Autodesk Fusion 360 part; units mm, degrees
note: some values were not read from the file. Set by a fixed rule: which sketch regions a step uses.
(part 5 of 8)
sketch "Sketch2" plane through (0, 0, 0) normal (0, 1, 0) x (1, 0, 0)
  spline S0 degree 3 poles (197.1624, -186.7544) (204.143, -186.8486) (204.2626, -186.9263) (213.6388, -187.2436) knots 0 0 0 0 1 1 1 1
  spline S1 degree 3 poles (213.6388, -187.2436) (214.883, -187.1742) (217.6529, -188.4891) (217.5074, -192.0215) knots 0 0 0 0 1 1 1 1
  spline S2 degree 3 poles (217.5074, -192.0215) (217.3575, -195.6649) (214.4757, -196.4537) (213.363, -196.3136) knots 0 0 0 0 1 1 1 1
  spline S3 degree 3 poles (213.363, -196.3136) (204.6057, -196.0144) (204.6194, -195.9201) (197.4444, -195.6721) knots 0 0 0 0 1 1 1 1
  spline S4 degree 3 poles (197.4444, -195.6721) (196.2085, -195.6886) (193.2735, -194.4066) (193.3889, -191.1038) knots 0 0 0 0 1 1 1 1
  spline S5 degree 3 poles (193.3889, -191.1038) (193.5215, -187.3144) (195.7446, -186.8906) (197.1624, -186.7544) knots 0 0 0 0 1 1 1 1
  spline S6 degree 3 poles (197.9086, -187.806) (199.8191, -187.8626) (201.0414, -189.5362) (201.0133, -191.0936) knots 0 0 0 0 1 1 1 1
  spline S7 degree 3 poles (201.0133, -191.0936) (200.9851, -192.7636) (199.4896, -194.3388) (197.734, -194.3215) knots 0 0 0 0 1 1 1 1
  spline S8 degree 3 poles (197.734, -194.3215) (196.0155, -194.305) (194.5332, -192.7609) (194.5124, -190.9876) knots 0 0 0 0 1 1 1 1
  spline S9 degree 3 poles (194.5124, -190.9876) (194.4922, -189.3414) (195.8726, -187.7455) (197.9086, -187.806) knots 0 0 0 0 1 1 1 1
  spline S10 degree 3 poles (197.835, -188.8319) (199.1587, -188.8732) (200.0057, -190.069) (199.9861, -191.1825) knots 0 0 0 0 1 1 1 1
  spline S11 degree 3 poles (199.9861, -191.1825) (199.9618, -192.3766) (198.9303, -193.5028) (197.7139, -193.4905) knots 0 0 0 0 1 1 1 1
  spline S12 degree 3 poles (197.7139, -193.4905) (196.5233, -193.4781) (195.4961, -192.3747) (195.4817, -191.1067) knots 0 0 0 0 1 1 1 1
  spline S13 degree 3 poles (195.4817, -191.1067) (195.4655, -189.9298) (196.4241, -188.7887) (197.835, -188.8319) knots 0 0 0 0 1 1 1 1
  spline S14 degree 3 poles (212.9182, -188.6603) (214.8287, -188.7169) (216.051, -190.3905) (216.0229, -191.9479) knots 0 0 0 0 1 1 1 1
  spline S15 degree 3 poles (216.0229, -191.9479) (215.9947, -193.6179) (214.4992, -195.1931) (212.7436, -195.1758) knots 0 0 0 0 1 1 1 1
  spline S16 degree 3 poles (212.7436, -195.1758) (211.0251, -195.1593) (209.5428, -193.6152) (209.522, -191.8419) knots 0 0 0 0 1 1 1 1
  spline S17 degree 3 poles (209.522, -191.8419) (209.5017, -190.1957) (210.8822, -188.5998) (212.9182, -188.6603) knots 0 0 0 0 1 1 1 1
  spline S18 degree 3 poles (212.8446, -189.6862) (214.1683, -189.7275) (215.0153, -190.9233) (214.9957, -192.0368) knots 0 0 0 0 1 1 1 1
  spline S19 degree 3 poles (214.9957, -192.0368) (214.9714, -193.2309) (213.9399, -194.3572) (212.7235, -194.3448) knots 0 0 0 0 1 1 1 1
  spline S20 degree 3 poles (212.7235, -194.3448) (211.5328, -194.3324) (210.5057, -193.229) (210.4913, -191.961) knots 0 0 0 0 1 1 1 1
  spline S21 degree 3 poles (210.4913, -191.961) (210.4751, -190.7841) (211.4337, -189.643) (212.8446, -189.6862) knots 0 0 0 0 1 1 1 1
  spline S22 degree 3 poles (197.838, -190.2751) (198.3138, -190.2875) (198.6181, -190.7091) (198.6111, -191.0999) knots 0 0 0 0 1 1 1 1
  spline S23 degree 3 poles (198.6111, -191.0999) (198.6029, -191.5188) (198.2317, -191.914) (197.7944, -191.9096) knots 0 0 0 0 1 1 1 1
  spline S24 degree 3 poles (197.7944, -191.9096) (197.3664, -191.9067) (196.9972, -191.5183) (196.9921, -191.0732) knots 0 0 0 0 1 1 1 1
  spline S25 degree 3 poles (196.9921, -191.0732) (196.9839, -190.6604) (197.331, -190.2599) (197.838, -190.2751) knots 0 0 0 0 1 1 1 1
  spline S26 degree 3 poles (212.8477, -191.1781) (213.3235, -191.1905) (213.6278, -191.6122) (213.6208, -192.0029) knots 0 0 0 0 1 1 1 1
  spline S27 degree 3 poles (213.6208, -192.0029) (213.6127, -192.4218) (213.2414, -192.817) (212.8041, -192.8127) knots 0 0 0 0 1 1 1 1
  spline S28 degree 3 poles (212.8041, -192.8127) (212.3761, -192.8097) (212.007, -192.4213) (212.0018, -191.9763) knots 0 0 0 0 1 1 1 1
  spline S29 degree 3 poles (212.0018, -191.9763) (211.9936, -191.5634) (212.3407, -191.163) (212.8477, -191.1781) knots 0 0 0 0 1 1 1 1
  line L0 (146.8173, -211.044) -> (145.571, -210.9331)
  spline S30 degree 3 poles (145.571, -210.9331) (143.4862, -215.1631) (142.3935, -219.9251) (142.4151, -224.6858) knots 0 0 0 0 1 1 1 1
  spline S31 degree 3 poles (142.4151, -224.6858) (142.4359, -229.2764) (143.4915, -233.8584) (145.4718, -237.9534) knots 0 0 0 0 1 1 1 1
  line L1 (145.4718, -237.9534) -> (146.4606, -237.8571)
  line L2 (146.4606, -237.8571) -> (147.0631, -234.8965)
  line L3 (147.0631, -234.8965) -> (150.0964, -235.1134)
  line L4 (150.0964, -235.1134) -> (150.3678, -238.2746)
  spline S32 degree 3 poles (150.3678, -238.2746) (151.1553, -238.2453) (151.9433, -238.2307) (152.7312, -238.2309) knots 0 0 0 0 1 1 1 1
  spline S33 degree 3 poles (152.7312, -238.2309) (154.9833, -238.2311) (157.2589, -238.3552) (159.4254, -238.9994) knots 0 0 0 0 1 1 1 1
  spline S34 degree 3 poles (159.4254, -238.9994) (162.7935, -240.0008) (165.7132, -242.1974) (168.9415, -243.6167) knots 0 0 0 0 1 1 1 1
  spline S35 degree 3 poles (168.9415, -243.6167) (172.5766, -245.2149) (176.5593, -245.8025) (180.5014, -245.825) knots 0 0 0 0 1 1 1 1
  spline S36 degree 3 poles (180.5014, -245.825) (184.2746, -245.8467) (188.086, -245.3531) (191.6142, -243.9513) knots 0 0 0 0 1 1 1 1
  spline S37 degree 3 poles (191.6142, -243.9513) (195.8272, -242.2775) (199.5984, -239.3333) (204.02, -238.4249) knots 0 0 0 0 1 1 1 1
  spline S38 degree 3 poles (204.02, -238.4249) (205.328, -238.1561) (206.6706, -238.0735) (207.9997, -238.1798) knots 0 0 0 0 1 1 1 1
  line L5 (207.9997, -238.1798) -> (210.3275, -238.3583)
  line L6 (210.3275, -238.3583) -> (210.7412, -235.154)
  line L7 (210.7412, -235.154) -> (213.4752, -235.2009)
  line L8 (213.4752, -235.2009) -> (213.9829, -237.8174)
  line L9 (213.9829, -237.8174) -> (215.6315, -237.7845)
  spline S39 degree 3 poles (215.6315, -237.7845) (216.1204, -236.7402) (216.5455, -235.6631) (216.9034, -234.562) knots 0 0 0 0 1 1 1 1
  spline S40 degree 3 poles (216.9034, -234.562) (217.9563, -231.3224) (218.4196, -227.8935) (218.4987, -224.4722) knots 0 0 0 0 1 1 1 1
  spline S41 degree 3 poles (218.4987, -224.4722) (218.5651, -221.6009) (218.3615, -218.7073) (217.6726, -215.9273) knots 0 0 0 0 1 1 1 1
  spline S42 degree 3 poles (217.6726, -215.9273) (217.2432, -214.1945) (216.6266, -212.5128) (215.8382, -210.9245) knots 0 0 0 0 1 1 1 1
  line L10 (215.8382, -210.9245) -> (214.0564, -210.9556)
  line L11 (214.0564, -210.9556) -> (213.8571, -214.0582)
  line L12 (213.8571, -214.0582) -> (210.5638, -213.8885)
  spline S43 degree 3 poles (210.5638, -213.8885) (210.5046, -213.3034) (210.4975, -212.7124) (210.5426, -212.1259) knots 0 0 0 0 1 1 1 1
  spline S44 degree 3 poles (210.5426, -212.1259) (210.56, -211.9007) (210.585, -211.6743) (210.5623, -211.4496) knots 0 0 0 0 1 1 1 1
  spline S45 degree 3 poles (210.5623, -211.4496) (210.5396, -211.225) (210.464, -210.9979) (210.3085, -210.8414) knots 0 0 0 0 1 1 1 1
  spline S46 degree 3 poles (210.3085, -210.8414) (210.1681, -210.7) (209.9673, -210.6272) (209.7735, -210.6474) knots 0 0 0 0 1 1 1 1
  spline S47 degree 3 poles (209.7735, -210.6474) (209.5798, -210.6676) (209.3966, -210.7805) (209.2855, -210.948) knots 0 0 0 0 1 1 1 1
  spline S48 degree 3 poles (209.2855, -210.948) (206.5352, -213.1438) (202.8342, -213.9747) (199.4667, -213.1524) knots 0 0 0 0 1 1 1 1
  spline S49 degree 3 poles (199.4667, -213.1524) (197.203, -212.5996) (195.155, -211.3642) (193.016, -210.4112) knots 0 0 0 0 1 1 1 1
  spline S50 degree 3 poles (193.016, -210.4112) (189.1059, -208.6692) (184.8324, -207.8633) (180.5841, -207.9409) knots 0 0 0 0 1 1 1 1
  spline S51 degree 3 poles (180.5841, -207.9409) (176.2965, -208.0192) (172.046, -208.9866) (168.0226, -210.5412) knots 0 0 0 0 1 1 1 1
  spline S52 degree 3 poles (168.0226, -210.5412) (164.8228, -211.7777) (161.6504, -213.4083) (158.2405, -213.4755) knots 0 0 0 0 1 1 1 1
  spline S53 degree 3 poles (158.2405, -213.4755) (156.4747, -213.5102) (154.6443, -213.0826) (153.26, -211.9336) knots 0 0 0 0 1 1 1 1
  spline S54 degree 3 poles (153.26, -211.9336) (152.9587, -211.6835) (152.6803, -211.4013) (152.3571, -211.1832) knots 0 0 0 0 1 1 1 1
  spline S55 degree 3 poles (152.3571, -211.1832) (152.0339, -210.9652) (151.6514, -210.8124) (151.2698, -210.8607) knots 0 0 0 0 1 1 1 1
  spline S56 degree 3 poles (151.2698, -210.8607) (150.972, -210.8984) (150.6905, -211.062) (150.5023, -211.3067) knots 0 0 0 0 1 1 1 1
  spline S57 degree 3 poles (150.5023, -211.3067) (150.3141, -211.5514) (150.2213, -211.8744) (150.2494, -212.1873) knots 0 0 0 0 1 1 1 1
  line L13 (150.2494, -212.1873) -> (150.145, -213.975)
  line L14 (150.145, -213.975) -> (146.911, -213.944)
  line L15 (146.911, -213.944) -> (146.8173, -211.044)
  line L16 (175.7107, -213.237) -> (185.3567, -213.3039)
  spline S58 degree 3 poles (185.3567, -213.3039) (185.5096, -213.2961) (185.6646, -213.358) (185.773, -213.4712) knots 0 0 0 0 1 1 1 1
  spline S59 degree 3 poles (185.773, -213.4712) (185.8812, -213.5842) (185.941, -213.7463) (185.9338, -213.9062) knots 0 0 0 0 1 1 1 1
  line L17 (185.9338, -213.9062) -> (185.9337, -235.3475)
  spline S60 degree 3 poles (185.9337, -235.3475) (185.9183, -235.5196) (185.8499, -235.686) (185.741, -235.8159) knots 0 0 0 0 1 1 1 1
  spline S61 degree 3 poles (185.741, -235.8159) (185.6255, -235.9539) (185.465, -236.0497) (185.2929, -236.0836) knots 0 0 0 0 1 1 1 1
  line L18 (185.2929, -236.0836) -> (175.7757, -235.8828)
  spline S62 degree 3 poles (175.7757, -235.8828) (175.6155, -235.8221) (175.4707, -235.7172) (175.36, -235.5816) knots 0 0 0 0 1 1 1 1
  spline S63 degree 3 poles (175.36, -235.5816) (175.2439, -235.4396) (175.1656, -235.2641) (175.1358, -235.0797) knots 0 0 0 0 1 1 1 1
  line L19 (175.1358, -235.0797) -> (175.104, -213.853)
  spline S64 degree 3 poles (175.104, -213.853) (175.1277, -213.7142) (175.1892, -213.5827) (175.2796, -213.4781) knots 0 0 0 0 1 1 1 1
  spline S65 degree 3 poles (175.2796, -213.4781) (175.3911, -213.349) (175.5463, -213.2622) (175.7107, -213.237) knots 0 0 0 0 1 1 1 1
  line L20 (163.8712, -228.7812) -> (163.868, -233.74)
  spline S66 degree 3 poles (163.868, -233.74) (163.8218, -234.0752) (163.931, -234.4301) (164.1552, -234.674) knots 0 0 0 0 1 1 1 1
  spline S67 degree 3 poles (164.1552, -234.674) (164.2785, -234.808) (164.4343, -234.909) (164.6038, -234.9647) knots 0 0 0 0 1 1 1 1
  spline S68 degree 3 poles (164.6038, -234.9647) (164.7733, -235.0204) (164.9562, -235.0307) (165.1304, -234.9943) knots 0 0 0 0 1 1 1 1
  line L21 (165.1304, -234.9943) -> (171.7879, -235.0398)
  spline S69 degree 3 poles (171.7879, -235.0398) (172.0447, -235.0158) (172.289, -234.8709) (172.4409, -234.6526) knots 0 0 0 0 1 1 1 1
  spline S70 degree 3 poles (172.4409, -234.6526) (172.5549, -234.4887) (172.6169, -234.2858) (172.615, -234.0831) knots 0 0 0 0 1 1 1 1
  line L22 (172.615, -234.0831) -> (172.6354, -228.7227)
  spline S71 degree 3 poles (172.6354, -228.7227) (172.6359, -228.5753) (172.6364, -228.4273) (172.6175, -228.2813) knots 0 0 0 0 1 1 1 1
  spline S72 degree 3 poles (172.6175, -228.2813) (172.5982, -228.1353) (172.5578, -227.99) (172.4801, -227.867) knots 0 0 0 0 1 1 1 1
  spline S73 degree 3 poles (172.4801, -227.867) (172.4091, -227.7546) (172.3076, -227.6636) (172.1907, -227.6073) knots 0 0 0 0 1 1 1 1
  spline S74 degree 3 poles (172.1907, -227.6073) (172.0737, -227.551) (171.9417, -227.5299) (171.814, -227.5467) knots 0 0 0 0 1 1 1 1
  line L23 (171.814, -227.5467) -> (164.537, -227.6136)
  spline S75 degree 3 poles (164.537, -227.6136) (164.3161, -227.6837) (164.121, -227.84) (163.9986, -228.045) knots 0 0 0 0 1 1 1 1
  spline S76 degree 3 poles (163.9986, -228.045) (163.8693, -228.2616) (163.8226, -228.5308) (163.8712, -228.7812) knots 0 0 0 0 1 1 1 1
  line L24 (187.8574, -228.9005) -> (187.94, -233.854)
  spline S77 degree 3 poles (187.94, -233.854) (187.9668, -234.1982) (188.1254, -234.5291) (188.3729, -234.7571) knots 0 0 0 0 1 1 1 1
  spline S78 degree 3 poles (188.3729, -234.7571) (188.596, -234.9627) (188.8888, -235.0835) (189.1858, -235.0924) knots 0 0 0 0 1 1 1 1
  line L25 (189.1858, -235.0924) -> (196.0238, -235.0728)
  spline S79 degree 3 poles (196.0238, -235.0728) (196.3427, -235.0628) (196.6527, -234.8824) (196.8289, -234.6037) knots 0 0 0 0 1 1 1 1
  spline S80 degree 3 poles (196.8289, -234.6037) (196.9017, -234.4886) (196.9517, -234.3584) (196.9788, -234.2233) knots 0 0 0 0 1 1 1 1
  spline S81 degree 3 poles (196.9788, -234.2233) (197.006, -234.0883) (197.009, -233.9494) (197.0096, -233.8114) knots 0 0 0 0 1 1 1 1
  line L26 (197.0096, -233.8114) -> (197.0283, -228.8335)
  spline S82 degree 3 poles (197.0283, -228.8335) (197.0087, -228.5255) (196.8648, -228.2282) (196.639, -228.0298) knots 0 0 0 0 1 1 1 1
  spline S83 degree 3 poles (196.639, -228.0298) (196.4425, -227.8572) (196.1867, -227.7603) (195.9303, -227.7614) knots 0 0 0 0 1 1 1 1
  line L27 (195.9303, -227.7614) -> (188.8433, -227.7337)
  spline S84 degree 3 poles (188.8433, -227.7337) (188.6771, -227.727) (188.5092, -227.7656) (188.3615, -227.8461) knots 0 0 0 0 1 1 1 1
  spline S85 degree 3 poles (188.3615, -227.8461) (188.2139, -227.9266) (188.0868, -228.048) (187.9969, -228.1947) knots 0 0 0 0 1 1 1 1
  spline S86 degree 3 poles (187.9969, -228.1947) (187.8702, -228.4014) (187.8195, -228.658) (187.8574, -228.9005) knots 0 0 0 0 1 1 1 1
  line L28 (169.9634, -222.2031) -> (162.7465, -223.073)
  spline S87 degree 3 poles (162.7465, -223.073) (162.475, -223.1042) (162.193, -223.0179) (161.9801, -222.8387) knots 0 0 0 0 1 1 1 1
  spline S88 degree 3 poles (161.9801, -222.8387) (161.8443, -222.7243) (161.7365, -222.5737) (161.6699, -222.405) knots 0 0 0 0 1 1 1 1
  spline S89 degree 3 poles (161.6699, -222.405) (161.6033, -222.2363) (161.5779, -222.0499) (161.5969, -221.8684) knots 0 0 0 0 1 1 1 1
  line L29 (161.5969, -221.8684) -> (161.4127, -219.6494)
  spline S90 degree 3 poles (161.4127, -219.6494) (161.3834, -219.4181) (161.4403, -219.1761) (161.5687, -218.9855) knots 0 0 0 0 1 1 1 1
  spline S91 degree 3 poles (161.5687, -218.9855) (161.7332, -218.7416) (162.0145, -218.5892) (162.2995, -218.5894) knots 0 0 0 0 1 1 1 1
  line L30 (162.2995, -218.5894) -> (169.261, -217.5857)
  spline S92 degree 3 poles (169.261, -217.5857) (169.5972, -217.5439) (169.9473, -217.6418) (170.219, -217.8533) knots 0 0 0 0 1 1 1 1
  spline S93 degree 3 poles (170.219, -217.8533) (170.5077, -218.0781) (170.7039, -218.4291) (170.7497, -218.8029) knots 0 0 0 0 1 1 1 1
  line L31 (170.7497, -218.8029) -> (170.8178, -220.9148)
  spline S94 degree 3 poles (170.8178, -220.9148) (170.8231, -221.2172) (170.7271, -221.5206) (170.5503, -221.7597) knots 0 0 0 0 1 1 1 1
  spline S95 degree 3 poles (170.5503, -221.7597) (170.4006, -221.9622) (170.1941, -222.1182) (169.9634, -222.2031) knots 0 0 0 0 1 1 1 1
  line L32 (198.1326, -223.2698) -> (191.2624, -221.8408)
  spline S96 degree 3 poles (191.2624, -221.8408) (190.9987, -221.7779) (190.7591, -221.6101) (190.6028, -221.3789) knots 0 0 0 0 1 1 1 1
  spline S97 degree 3 poles (190.6028, -221.3789) (190.4019, -221.0819) (190.3456, -220.6832) (190.4556, -220.3379) knots 0 0 0 0 1 1 1 1
  line L33 (190.4556, -220.3379) -> (190.7601, -218.1736)
  spline S98 degree 3 poles (190.7601, -218.1736) (190.7759, -217.95) (190.8819, -217.735) (191.0468, -217.5921) knots 0 0 0 0 1 1 1 1
  spline S99 degree 3 poles (191.0468, -217.5921) (191.1507, -217.5021) (191.2767, -217.4404) (191.4093, -217.4147) knots 0 0 0 0 1 1 1 1
  spline S100 degree 3 poles (191.4093, -217.4147) (191.5419, -217.389) (191.6807, -217.3993) (191.8084, -217.4444) knots 0 0 0 0 1 1 1 1
  line L34 (191.8084, -217.4444) -> (198.4707, -218.6665)
  spline S101 degree 3 poles (198.4707, -218.6665) (198.7976, -218.7419) (199.0971, -218.9416) (199.3006, -219.22) knots 0 0 0 0 1 1 1 1
  spline S102 degree 3 poles (199.3006, -219.22) (199.5205, -219.5206) (199.6258, -219.9106) (199.5888, -220.2874) knots 0 0 0 0 1 1 1 1
  line L35 (199.5888, -220.2874) -> (199.1997, -222.3137)
  spline S103 degree 3 poles (199.1997, -222.3137) (199.1469, -222.5972) (198.9912, -222.8583) (198.7711, -223.0322) knots 0 0 0 0 1 1 1 1
  spline S104 degree 3 poles (198.7711, -223.0322) (198.5879, -223.1769) (198.3618, -223.261) (198.1326, -223.2698) knots 0 0 0 0 1 1 1 1
  spline S105 degree 3 poles (177.8346, -243.1583) (177.9569, -243.2502) (178.0973, -243.3149) (178.2439, -243.3509) knots 0 0 0 0 1 1 1 1
  spline S106 degree 3 poles (178.2439, -243.3509) (178.3905, -243.3868) (178.5421, -243.3925) (178.6926, -243.395) knots 0 0 0 0 1 1 1 1
  line L36 (178.6926, -243.395) -> (181.7935, -243.4438)
  spline S107 degree 3 poles (181.7935, -243.4438) (182.1582, -243.4314) (182.5153, -243.2555) (182.7571, -242.9691) knots 0 0 0 0 1 1 1 1
  spline S108 degree 3 poles (182.7571, -242.9691) (183.012, -242.6672) (183.1342, -242.2452) (183.0758, -241.8468) knots 0 0 0 0 1 1 1 1
  spline S109 degree 3 poles (183.0758, -241.8468) (183.0174, -241.4483) (182.7778, -241.082) (182.441, -240.8871) knots 0 0 0 0 1 1 1 1
  spline S110 degree 3 poles (182.441, -240.8871) (182.1958, -240.7452) (181.9039, -240.6943) (181.6281, -240.7451) knots 0 0 0 0 1 1 1 1
  line L37 (181.6281, -240.7451) -> (178.6145, -240.6969)
  spline S111 degree 3 poles (178.6145, -240.6969) (178.4687, -240.6946) (178.3213, -240.6973) (178.1801, -240.7352) knots 0 0 0 0 1 1 1 1
  spline S112 degree 3 poles (178.1801, -240.7352) (178.0388, -240.773) (177.9062, -240.8429) (177.7894, -240.9344) knots 0 0 0 0 1 1 1 1
  spline S113 degree 3 poles (177.7894, -240.9344) (177.4586, -241.1938) (177.2577, -241.6257) (177.2665, -242.0586) knots 0 0 0 0 1 1 1 1
  spline S114 degree 3 poles (177.2665, -242.0586) (177.2749, -242.4914) (177.4935, -242.9139) (177.8346, -243.1583) knots 0 0 0 0 1 1 1 1
  spline S115 degree 3 poles (180.2732, -237.6694) (180.0071, -237.6806) (179.7202, -238.0057) (179.7313, -238.2845) knots 0 0 0 0 1 1 1 1
  spline S116 degree 3 poles (179.7313, -238.2845) (179.7419, -238.541) (180.0282, -238.8055) (180.2732, -238.805) knots 0 0 0 0 1 1 1 1
  spline S117 degree 3 poles (180.2732, -238.805) (180.5395, -238.8045) (180.8603, -238.5163) (180.8603, -238.2372) knots 0 0 0 0 1 1 1 1
  spline S118 degree 3 poles (180.8603, -238.2372) (180.8603, -237.9581) (180.5393, -237.6582) (180.2732, -237.6694) knots 0 0 0 0 1 1 1 1
  spline S119 degree 3 poles (180.5218, -210.2723) (180.2557, -210.2835) (179.9688, -210.6087) (179.9799, -210.8875) knots 0 0 0 0 1 1 1 1
  spline S120 degree 3 poles (179.9799, -210.8875) (179.9904, -211.144) (180.2767, -211.4084) (180.5218, -211.408) knots 0 0 0 0 1 1 1 1
  spline S121 degree 3 poles (180.5218, -211.408) (180.7881, -211.4075) (181.1088, -211.1192) (181.1088, -210.8401) knots 0 0 0 0 1 1 1 1
  spline S122 degree 3 poles (181.1088, -210.8401) (181.1088, -210.5611) (180.7879, -210.2612) (180.5218, -210.2723) knots 0 0 0 0 1 1 1 1
  spline S123 degree 3 poles (87.8092, -110.5513) (84.4644, -110.7337) (81.2096, -112.3316) (78.976, -114.9054) knots 0 0 0 0 1 1 1 1
  spline S124 degree 3 poles (78.976, -114.9054) (76.7424, -117.4793) (75.5617, -120.999) (75.7923, -124.4447) knots 0 0 0 0 1 1 1 1
  spline S125 degree 3 poles (75.7923, -124.4447) (76.0144, -127.7646) (77.5393, -130.9695) (79.9391, -133.1945) knots 0 0 0 0 1 1 1 1
  spline S126 degree 3 poles (79.9391, -133.1945) (82.3389, -135.4195) (85.5846, -136.6429) (88.8106, -136.5545) knots 0 0 0 0 1 1 1 1
  spline S127 degree 3 poles (88.8106, -136.5545) (92.0915, -136.4647) (95.3217, -135.0173) (97.6124, -132.5937) knots 0 0 0 0 1 1 1 1
  spline S128 degree 3 poles (97.6124, -132.5937) (99.9031, -130.1702) (101.2243, -126.7962) (101.1918, -123.4121) knots 0 0 0 0 1 1 1 1
  spline S129 degree 3 poles (101.1918, -123.4121) (101.158, -119.8994) (99.6612, -116.4302) (97.1652, -114.0394) knots 0 0 0 0 1 1 1 1
  spline S130 degree 3 poles (97.1652, -114.0394) (94.6692, -111.6487) (91.2112, -110.3658) (87.8092, -110.5513) knots 0 0 0 0 1 1 1 1
  line L38 (84.4864, -120.8306) -> (80.3552, -118.6188)
  spline S131 degree 3 poles (80.3552, -118.6188) (80.0541, -118.3839) (79.8577, -118.0117) (79.8299, -117.6234) knots 0 0 0 0 1 1 1 1
  spline S132 degree 3 poles (79.8299, -117.6234) (79.8021, -117.2352) (79.9433, -116.8373) (80.2076, -116.5593) knots 0 0 0 0 1 1 1 1
  spline S133 degree 3 poles (80.2076, -116.5593) (80.4641, -116.2894) (80.8323, -116.1363) (81.1986, -116.1473) knots 0 0 0 0 1 1 1 1
  spline S134 degree 3 poles (81.1986, -116.1473) (81.5649, -116.1583) (81.9239, -116.3329) (82.1649, -116.6176) knots 0 0 0 0 1 1 1 1
  line L39 (82.1649, -116.6176) -> (84.8827, -120.2827)
  spline S135 degree 3 poles (84.8827, -120.2827) (84.932, -120.3278) (84.9679, -120.3882) (84.9844, -120.454) knots 0 0 0 0 1 1 1 1
  spline S136 degree 3 poles (84.9844, -120.454) (85.0008, -120.5198) (84.9978, -120.5906) (84.9756, -120.6545) knots 0 0 0 0 1 1 1 1
  spline S137 degree 3 poles (84.9756, -120.6545) (84.9424, -120.7508) (84.8654, -120.8298) (84.7718, -120.8634) knots 0 0 0 0 1 1 1 1
  spline S138 degree 3 poles (84.7718, -120.8634) (84.6783, -120.897) (84.5703, -120.8847) (84.4864, -120.8306) knots 0 0 0 0 1 1 1 1
  spline S139 degree 3 poles (95.6202, -128.158) (95.9132, -128.3374) (96.1338, -128.6384) (96.2211, -128.9781) knots 0 0 0 0 1 1 1 1
  spline S140 degree 3 poles (96.2211, -128.9781) (96.3084, -129.3177) (96.2613, -129.6919) (96.0929, -129.9974) knots 0 0 0 0 1 1 1 1
  spline S141 degree 3 poles (96.0929, -129.9974) (95.8981, -130.3507) (95.5421, -130.6046) (95.1527, -130.6679) knots 0 0 0 0 1 1 1 1
  spline S142 degree 3 poles (95.1527, -130.6679) (94.7634, -130.7312) (94.3488, -130.6024) (94.0581, -130.328) knots 0 0 0 0 1 1 1 1
  line L40 (94.0581, -130.328) -> (91.2245, -126.6641)
  spline S143 degree 3 poles (91.2245, -126.6641) (91.1733, -126.6007) (91.1442, -126.5188) (91.1434, -126.4364) knots 0 0 0 0 1 1 1 1
  spline S144 degree 3 poles (91.1434, -126.4364) (91.1427, -126.3539) (91.1704, -126.2715) (91.2204, -126.2072) knots 0 0 0 0 1 1 1 1
  spline S145 degree 3 poles (91.2204, -126.2072) (91.2797, -126.1309) (91.3703, -126.0812) (91.4648, -126.0732) knots 0 0 0 0 1 1 1 1
  spline S146 degree 3 poles (91.4648, -126.0732) (91.5593, -126.0655) (91.6565, -126.0987) (91.7272, -126.164) knots 0 0 0 0 1 1 1 1
  line L41 (91.7272, -126.164) -> (95.6202, -128.158)
  spline S147 degree 3 poles (95.9599, -119.2214) (96.2252, -119.0218) (96.5745, -118.9456) (96.8954, -119.0173) knots 0 0 0 0 1 1 1 1
  spline S148 degree 3 poles (96.8954, -119.0173) (97.2164, -119.089) (97.5038, -119.3074) (97.6652, -119.6023) knots 0 0 0 0 1 1 1 1
  spline S149 degree 3 poles (97.6652, -119.6023) (97.8241, -119.8927) (97.8586, -120.2527) (97.7577, -120.5695) knots 0 0 0 0 1 1 1 1
  spline S150 degree 3 poles (97.7577, -120.5695) (97.6569, -120.8864) (97.4224, -121.1553) (97.1275, -121.2922) knots 0 0 0 0 1 1 1 1
  line L42 (97.1275, -121.2922) -> (92.6606, -122.3661)
  spline S151 degree 3 poles (92.6606, -122.3661) (92.5844, -122.3932) (92.4995, -122.3932) (92.4234, -122.366) knots 0 0 0 0 1 1 1 1
  spline S152 degree 3 poles (92.4234, -122.366) (92.3472, -122.3388) (92.2805, -122.2847) (92.2369, -122.2148) knots 0 0 0 0 1 1 1 1
  spline S153 degree 3 poles (92.2369, -122.2148) (92.1932, -122.1447) (92.1731, -122.0593) (92.181, -121.9763) knots 0 0 0 0 1 1 1 1
  spline S154 degree 3 poles (92.181, -121.9763) (92.1888, -121.8935) (92.2244, -121.8135) (92.2803, -121.7534) knots 0 0 0 0 1 1 1 1
  line L43 (92.2803, -121.7534) -> (95.9599, -119.2214)
  spline S155 degree 3 poles (80.0727, -128.0707) (79.7927, -128.1901) (79.4687, -128.1952) (79.1853, -128.0848) knots 0 0 0 0 1 1 1 1
  spline S156 degree 3 poles (79.1853, -128.0848) (78.9018, -127.9744) (78.662, -127.7496) (78.5285, -127.4691) knots 0 0 0 0 1 1 1 1
  spline S157 degree 3 poles (78.5285, -127.4691) (78.3753, -127.1472) (78.3661, -126.7559) (78.5042, -126.4268) knots 0 0 0 0 1 1 1 1
  spline S158 degree 3 poles (78.5042, -126.4268) (78.6423, -126.0976) (78.9251, -125.8366) (79.2575, -125.7313) knots 0 0 0 0 1 1 1 1
  line L44 (79.2575, -125.7313) -> (83.8162, -124.7898)
  spline S159 degree 3 poles (83.8162, -124.7898) (83.8943, -124.753) (83.9857, -124.7472) (84.0675, -124.774) knots 0 0 0 0 1 1 1 1
  spline S160 degree 3 poles (84.0675, -124.774) (84.1493, -124.8007) (84.2207, -124.8599) (84.2639, -124.9364) knots 0 0 0 0 1 1 1 1
  spline S161 degree 3 poles (84.2639, -124.9364) (84.3074, -125.0137) (84.3216, -125.108) (84.3028, -125.1953) knots 0 0 0 0 1 1 1 1
  spline S162 degree 3 poles (84.3028, -125.1953) (84.2841, -125.2826) (84.2325, -125.3618) (84.1614, -125.4129) knots 0 0 0 0 1 1 1 1
  line L45 (84.1614, -125.4129) -> (80.0727, -128.0707)
  line L46 (88.6675, -119.2132) -> (88.6462, -114.3656)
  spline S163 degree 3 poles (88.6462, -114.3656) (88.6118, -114.0183) (88.7286, -113.658) (88.9586, -113.4017) knots 0 0 0 0 1 1 1 1
  spline S164 degree 3 poles (88.9586, -113.4017) (89.1886, -113.1455) (89.528, -112.9976) (89.8665, -113.0061) knots 0 0 0 0 1 1 1 1
  spline S165 degree 3 poles (89.8665, -113.0061) (90.2609, -113.016) (90.6443, -113.2416) (90.8531, -113.5868) knots 0 0 0 0 1 1 1 1
  spline S166 degree 3 poles (90.8531, -113.5868) (91.062, -113.9319) (91.0901, -114.3861) (90.9253, -114.7558) knots 0 0 0 0 1 1 1 1
  line L47 (90.9253, -114.7558) -> (89.4733, -119.3472)
  spline S167 degree 3 poles (89.4733, -119.3472) (89.4555, -119.4444) (89.4032, -119.5345) (89.3285, -119.5966) knots 0 0 0 0 1 1 1 1
  spline S168 degree 3 poles (89.3285, -119.5966) (89.2538, -119.6587) (89.1574, -119.6924) (89.0614, -119.6899) knots 0 0 0 0 1 1 1 1
  spline S169 degree 3 poles (89.0614, -119.6899) (88.9473, -119.6866) (88.8355, -119.6316) (88.7614, -119.5421) knots 0 0 0 0 1 1 1 1
  spline S170 degree 3 poles (88.7614, -119.5421) (88.6874, -119.4525) (88.6523, -119.3299) (88.6675, -119.2132) knots 0 0 0 0 1 1 1 1
  spline S171 degree 3 poles (87.8691, -127.9185) (87.8804, -129.4278) (87.8877, -130.937) (87.891, -132.4463) knots 0 0 0 0 1 1 1 1
  spline S172 degree 3 poles (87.891, -132.4463) (87.8988, -132.7851) (87.7649, -133.1249) (87.5302, -133.3622) knots 0 0 0 0 1 1 1 1
  spline S173 degree 3 poles (87.5302, -133.3622) (87.2955, -133.5995) (86.9633, -133.7308) (86.635, -133.7161) knots 0 0 0 0 1 1 1 1
  spline S174 degree 3 poles (86.635, -133.7161) (86.264, -133.6995) (85.9053, -133.4946) (85.6949, -133.1791) knots 0 0 0 0 1 1 1 1
  spline S175 degree 3 poles (85.6949, -133.1791) (85.4845, -132.8636) (85.4274, -132.445) (85.5451, -132.0818) knots 0 0 0 0 1 1 1 1
  line L48 (85.5451, -132.0818) -> (87.0396, -127.7934)
  spline S176 degree 3 poles (87.0396, -127.7934) (87.0646, -127.6994) (87.1212, -127.6147) (87.1975, -127.5571) knots 0 0 0 0 1 1 1 1
  spline S177 degree 3 poles (87.1975, -127.5571) (87.2738, -127.4995) (87.3692, -127.4695) (87.4636, -127.4733) knots 0 0 0 0 1 1 1 1
  spline S178 degree 3 poles (87.4636, -127.4733) (87.5729, -127.4777) (87.6798, -127.528) (87.7547, -127.6103) knots 0 0 0 0 1 1 1 1
  spline S179 degree 3 poles (87.7547, -127.6103) (87.8296, -127.6925) (87.8716, -127.8056) (87.8691, -127.9185) knots 0 0 0 0 1 1 1 1
  spline S180 degree 3 poles (88.269, -123.108) (88.146, -123.1002) (88.0207, -123.1465) (87.9306, -123.2331) knots 0 0 0 0 1 1 1 1
  spline S181 degree 3 poles (87.9306, -123.2331) (87.8405, -123.3198) (87.787, -123.4456) (87.7862, -123.5726) knots 0 0 0 0 1 1 1 1
  spline S182 degree 3 poles (87.7862, -123.5726) (87.7854, -123.6839) (87.8247, -123.795) (87.8949, -123.8796) knots 0 0 0 0 1 1 1 1
  spline S183 degree 3 poles (87.8949, -123.8796) (87.9651, -123.9642) (88.0656, -124.0214) (88.1724, -124.0373) knots 0 0 0 0 1 1 1 1
  spline S184 degree 3 poles (88.1724, -124.0373) (88.3005, -124.0563) (88.4358, -124.0147) (88.5332, -123.9268) knots 0 0 0 0 1 1 1 1
  spline S185 degree 3 poles (88.5332, -123.9268) (88.6305, -123.8388) (88.6882, -123.7061) (88.6874, -123.5726) knots 0 0 0 0 1 1 1 1
  spline S186 degree 3 poles (88.6874, -123.5726) (88.6867, -123.4566) (88.6425, -123.3413) (88.5659, -123.2563) knots 0 0 0 0 1 1 1 1
  spline S187 degree 3 poles (88.5659, -123.2563) (88.4893, -123.1712) (88.3812, -123.1172) (88.269, -123.108) knots 0 0 0 0 1 1 1 1
  line L49 (145.2117, -33.5799) -> (147.4066, -33.5799)
  line L50 (147.4066, -33.5799) -> (147.4066, -34.5824)
  spline S188 degree 3 poles (147.4066, -34.5824) (147.3948, -34.6957) (147.4282, -34.813) (147.498, -34.9031) knots 0 0 0 0 1 1 1 1
  spline S189 degree 3 poles (147.498, -34.9031) (147.5825, -35.0122) (147.7197, -35.0787) (147.8578, -35.0775) knots 0 0 0 0 1 1 1 1
  line L51 (147.8578, -35.0775) -> (150.9272, -35.0693)
  spline S190 degree 3 poles (150.9272, -35.0693) (151.0916, -35.0681) (151.2548, -35.005) (151.377, -34.8949) knots 0 0 0 0 1 1 1 1
  spline S191 degree 3 poles (151.377, -34.8949) (151.5109, -34.7747) (151.5937, -34.5991) (151.6017, -34.4195) knots 0 0 0 0 1 1 1 1
  line L52 (151.6017, -34.4195) -> (151.583, -33.5673)
  line L53 (151.583, -33.5673) -> (153.2135, -33.5306)
  line L54 (153.2135, -33.5306) -> (154.9512, -39.4744)
  line L55 (154.9512, -39.4744) -> (140.4097, -39.4019)
  line L56 (140.4097, -39.4019) -> (145.2113, -33.5784)
  line L57 (145.2113, -33.5784) -> (145.2117, -33.5799)
  spline S192 degree 3 poles (152.8917, -139.0521) (153.0078, -138.4957) (152.8191, -137.9022) (152.3857, -137.4605) knots 0 0 0 0 1 1 1 1
  spline S193 degree 3 poles (152.3857, -137.4605) (152.0239, -137.0918) (151.4979, -136.8313) (150.9281, -136.7386) knots 0 0 0 0 1 1 1 1
  line L58 (150.9281, -136.7386) -> (134.6913, -136.4064)
  spline S194 degree 3 poles (134.6913, -136.4064) (134.146, -136.347) (133.5728, -136.4832) (133.1531, -136.7716) knots 0 0 0 0 1 1 1 1
  spline S195 degree 3 poles (133.1531, -136.7716) (132.8925, -136.9507) (132.6908, -137.1857) (132.5743, -137.4461) knots 0 0 0 0 1 1 1 1
  spline S196 degree 3 poles (132.5743, -137.4461) (132.4578, -137.7065) (132.4268, -137.9916) (132.4852, -138.2646) knots 0 0 0 0 1 1 1 1
  line L59 (132.4852, -138.2646) -> (128.5982, -202.0579)
  spline S197 degree 3 poles (128.5982, -202.0579) (128.6214, -202.6789) (128.8788, -203.293) (129.3272, -203.797) knots 0 0 0 0 1 1 1 1
  spline S198 degree 3 poles (129.3272, -203.797) (129.8039, -204.333) (130.4952, -204.7415) (131.2705, -204.9456) knots 0 0 0 0 1 1 1 1
  line L60 (131.2705, -204.9456) -> (185.2831, -208.4897)
  spline S199 degree 3 poles (185.2831, -208.4897) (186.4596, -208.6439) (187.7184, -208.3018) (188.5423, -207.6038) knots 0 0 0 0 1 1 1 1
  spline S200 degree 3 poles (188.5423, -207.6038) (189.0223, -207.1971) (189.3564, -206.6786) (189.4939, -206.127) knots 0 0 0 0 1 1 1 1
  spline S201 degree 3 poles (189.4939, -206.127) (191.7707, -198.9053) (192.2145, -191.3074) (190.7896, -183.9437) knots 0 0 0 0 1 1 1 1
  spline S202 degree 3 poles (190.7896, -183.9437) (190.5261, -182.5822) (190.1911, -181.2078) (189.4212, -179.979) knots 0 0 0 0 1 1 1 1
  spline S203 degree 3 poles (189.4212, -179.979) (189.0363, -179.3645) (188.5431, -178.7911) (187.9294, -178.3141) knots 0 0 0 0 1 1 1 1
  spline S204 degree 3 poles (187.9294, -178.3141) (187.3158, -177.8372) (186.5791, -177.4584) (185.7689, -177.2493) knots 0 0 0 0 1 1 1 1
  spline S205 degree 3 poles (185.7689, -177.2493) (184.7384, -176.9834) (183.6227, -176.9987) (182.5591, -177.1574) knots 0 0 0 0 1 1 1 1
  spline S206 degree 3 poles (182.5591, -177.1574) (181.4955, -177.3161) (180.472, -177.613) (179.4526, -177.9056) knots 0 0 0 0 1 1 1 1
  spline S207 degree 3 poles (179.4526, -177.9056) (174.0534, -179.4552) (168.6158, -180.9152) (163.176, -182.3685) knots 0 0 0 0 1 1 1 1
  spline S208 degree 3 poles (163.176, -182.3685) (161.7568, -182.7477) (160.3289, -183.1281) (158.8509, -183.3067) knots 0 0 0 0 1 1 1 1
  spline S209 degree 3 poles (158.8509, -183.3067) (157.3729, -183.4852) (155.8279, -183.4535) (154.4303, -183.0248) knots 0 0 0 0 1 1 1 1
  spline S210 degree 3 poles (154.4303, -183.0248) (153.2607, -182.6661) (152.2165, -182.0263) (151.515, -181.1873) knots 0 0 0 0 1 1 1 1
  spline S211 degree 3 poles (151.515, -181.1873) (150.6897, -180.2002) (150.3628, -178.9477) (150.6243, -177.7744) knots 0 0 0 0 1 1 1 1
  line L61 (150.6243, -177.7744) -> (152.8917, -139.0521)
  line L62 (141.7632, -151.1039) -> (144.1108, -148.9227)
  spline S212 degree 3 poles (144.1108, -148.9227) (144.2958, -148.6887) (144.3545, -148.3916) (144.2688, -148.1225) knots 0 0 0 0 1 1 1 1
  spline S213 degree 3 poles (144.2688, -148.1225) (144.1831, -147.8534) (143.9544, -147.6163) (143.6528, -147.4841) knots 0 0 0 0 1 1 1 1
  spline S214 degree 3 poles (143.6528, -147.4841) (143.3009, -147.3298) (142.8561, -147.324) (142.4982, -147.469) knots 0 0 0 0 1 1 1 1
  spline S215 degree 3 poles (142.4982, -147.469) (142.1404, -147.614) (141.8793, -147.9059) (141.8204, -148.2266) knots 0 0 0 0 1 1 1 1
  spline S216 degree 3 poles (141.8204, -148.2266) (141.803, -148.0666) (141.7347, -147.9104) (141.6242, -147.777) knots 0 0 0 0 1 1 1 1
  spline S217 degree 3 poles (141.6242, -147.777) (141.5137, -147.6436) (141.3611, -147.5333) (141.1849, -147.4596) knots 0 0 0 0 1 1 1 1
  spline S218 degree 3 poles (141.1849, -147.4596) (141.0087, -147.386) (140.8094, -147.349) (140.6112, -147.3532) knots 0 0 0 0 1 1 1 1
  spline S219 degree 3 poles (140.6112, -147.3532) (140.4131, -147.3572) (140.2164, -147.4029) (140.0454, -147.4841) knots 0 0 0 0 1 1 1 1
  spline S220 degree 3 poles (140.0454, -147.4841) (139.755, -147.6218) (139.5436, -147.8645) (139.4809, -148.1324) knots 0 0 0 0 1 1 1 1
  spline S221 degree 3 poles (139.4809, -148.1324) (139.4181, -148.4003) (139.5049, -148.6889) (139.7127, -148.9033) knots 0 0 0 0 1 1 1 1
  line L63 (139.7127, -148.9033) -> (141.7632, -151.1039)
  spline S222 degree 3 poles (172.6908, -194.5103) (172.8746, -194.4232) (173.0234, -194.2884) (173.1099, -194.1307) knots 0 0 0 0 1 1 1 1
  spline S223 degree 3 poles (173.1099, -194.1307) (173.1963, -193.973) (173.22, -193.7932) (173.1767, -193.6243) knots 0 0 0 0 1 1 1 1
  spline S224 degree 3 poles (173.1767, -193.6243) (173.133, -193.4541) (173.0214, -193.2959) (172.8627, -193.1789) knots 0 0 0 0 1 1 1 1
  spline S225 degree 3 poles (172.8627, -193.1789) (172.704, -193.062) (172.499, -192.9871) (172.2859, -192.968) knots 0 0 0 0 1 1 1 1
  line L64 (172.2859, -192.968) -> (161.4753, -190.7365)
  spline S226 degree 3 poles (161.4753, -190.7365) (161.2286, -190.6886) (160.9657, -190.6968) (160.7244, -190.7601) knots 0 0 0 0 1 1 1 1
  spline S227 degree 3 poles (160.7244, -190.7601) (160.483, -190.8234) (160.2639, -190.9415) (160.0987, -191.0975) knots 0 0 0 0 1 1 1 1
  spline S228 degree 3 poles (160.0987, -191.0975) (159.923, -191.2633) (159.8089, -191.4713) (159.7747, -191.6881) knots 0 0 0 0 1 1 1 1
  line L65 (159.7747, -191.6881) -> (159.6938, -197.0289)
  spline S229 degree 3 poles (159.6938, -197.0289) (159.7082, -197.3747) (159.9506, -197.7088) (160.3163, -197.8872) knots 0 0 0 0 1 1 1 1
  spline S230 degree 3 poles (160.3163, -197.8872) (160.5144, -197.9838) (160.7451, -198.036) (160.9763, -198.0365) knots 0 0 0 0 1 1 1 1
  spline S231 degree 3 poles (160.9763, -198.0365) (161.2075, -198.037) (161.4385, -197.9858) (161.6373, -197.8901) knots 0 0 0 0 1 1 1 1
  line L66 (161.6373, -197.8901) -> (172.6908, -194.5103)
  spline S232 degree 3 poles (134.1641, -194.3951) (135, -194.7407) (135.9621, -194.8188) (136.8996, -194.8522) knots 0 0 0 0 1 1 1 1
  spline S233 degree 3 poles (136.8996, -194.8522) (137.5374, -194.8749) (138.1761, -194.8798) (138.8143, -194.8668) knots 0 0 0 0 1 1 1 1
  line L67 (138.8143, -194.8668) -> (139.6732, -193.8922)
  line L68 (139.6732, -193.8922) -> (140.5034, -194.9596)
  spline S234 degree 3 poles (140.5034, -194.9596) (142.422, -194.9722) (144.3409, -194.949) (146.2581, -194.8899) knots 0 0 0 0 1 1 1 1
  spline S235 degree 3 poles (146.2581, -194.8899) (147.4759, -194.8524) (148.6979, -194.8001) (149.8941, -194.6115) knots 0 0 0 0 1 1 1 1
  spline S236 degree 3 poles (149.8941, -194.6115) (151.0608, -194.4276) (152.2179, -194.105) (153.1586, -193.5162) knots 0 0 0 0 1 1 1 1
  spline S237 degree 3 poles (153.1586, -193.5162) (153.4604, -193.3273) (153.7461, -193.1024) (153.8836, -192.8141) knots 0 0 0 0 1 1 1 1
  spline S238 degree 3 poles (153.8836, -192.8141) (153.9523, -192.6699) (153.9814, -192.5118) (153.9523, -192.3591) knots 0 0 0 0 1 1 1 1
  spline S239 degree 3 poles (153.9523, -192.3591) (153.9232, -192.2063) (153.8338, -192.0596) (153.6916, -191.9566) knots 0 0 0 0 1 1 1 1
  spline S240 degree 3 poles (153.6916, -191.9566) (153.522, -191.8338) (153.2801, -191.7798) (153.0568, -191.8149) knots 0 0 0 0 1 1 1 1
  line L69 (153.0568, -191.8149) -> (151.0353, -191.9187)
  line L70 (151.0353, -191.9187) -> (150.9871, -190.6192)
  line L71 (150.9871, -190.6192) -> (150.3275, -190.313)
  spline S241 degree 3 poles (150.3275, -190.313) (150.204, -190.2897) (150.0698, -190.3061) (149.9598, -190.3568) knots 0 0 0 0 1 1 1 1
  spline S242 degree 3 poles (149.9598, -190.3568) (149.8138, -190.4246) (149.7148, -190.5544) (149.7051, -190.6905) knots 0 0 0 0 1 1 1 1
  line L72 (149.7051, -190.6905) -> (149.78, -192.5463)
  line L73 (149.78, -192.5463) -> (147.6217, -192.5599)
  line L74 (147.6217, -192.5599) -> (147.5329, -191.3622)
  line L75 (147.5329, -191.3622) -> (147.2324, -191.1113)
  spline S243 degree 3 poles (147.2324, -191.1113) (147.1579, -191.049) (147.0854, -190.9849) (147.0044, -190.9281) knots 0 0 0 0 1 1 1 1
  spline S244 degree 3 poles (147.0044, -190.9281) (146.9234, -190.8715) (146.8288, -190.8229) (146.7228, -190.8106) knots 0 0 0 0 1 1 1 1
  spline S245 degree 3 poles (146.7228, -190.8106) (146.6699, -190.8048) (146.615, -190.8077) (146.5644, -190.8219) knots 0 0 0 0 1 1 1 1
  spline S246 degree 3 poles (146.5644, -190.8219) (146.5137, -190.836) (146.4678, -190.8609) (146.4322, -190.8933) knots 0 0 0 0 1 1 1 1
  spline S247 degree 3 poles (146.4322, -190.8933) (146.3965, -190.9256) (146.3715, -190.9651) (146.3558, -191.0066) knots 0 0 0 0 1 1 1 1
  spline S248 degree 3 poles (146.3558, -191.0066) (146.3402, -191.048) (146.3338, -191.0913) (146.3278, -191.1345) knots 0 0 0 0 1 1 1 1
  line L76 (146.3278, -191.1345) -> (146.2905, -191.4086)
  line L77 (146.2905, -191.4086) -> (146.222, -192.6447)
  line L78 (146.222, -192.6447) -> (143.6817, -192.6267)
  line L79 (143.6817, -192.6267) -> (143.5874, -191.2445)
  spline S249 degree 3 poles (143.5874, -191.2445) (143.6023, -191.1578) (143.5727, -191.0666) (143.5067, -190.9972) knots 0 0 0 0 1 1 1 1
  spline S250 degree 3 poles (143.5067, -190.9972) (143.4409, -190.9278) (143.3398, -190.8811) (143.2326, -190.8705) knots 0 0 0 0 1 1 1 1
  spline S251 degree 3 poles (143.2326, -190.8705) (143.1415, -190.8617) (143.0483, -190.8774) (142.9644, -190.9081) knots 0 0 0 0 1 1 1 1
  spline S252 degree 3 poles (142.9644, -190.9081) (142.8804, -190.9384) (142.8049, -190.9821) (142.734, -191.0295) knots 0 0 0 0 1 1 1 1
  spline S253 degree 3 poles (142.734, -191.0295) (142.5693, -191.1392) (142.426, -191.2699) (142.3109, -191.4154) knots 0 0 0 0 1 1 1 1
  line L80 (142.3109, -191.4154) -> (142.2083, -192.4994)
  line L81 (142.2083, -192.4994) -> (141.5281, -192.4886)
  spline S254 degree 3 poles (141.5281, -192.4886) (141.4869, -192.1385) (141.3109, -191.7996) (141.0307, -191.531) knots 0 0 0 0 1 1 1 1
  spline S255 degree 3 poles (141.0307, -191.531) (140.7506, -191.2624) (140.3675, -191.0654) (139.9484, -190.9742) knots 0 0 0 0 1 1 1 1
  spline S256 degree 3 poles (139.9484, -190.9742) (139.3735, -190.8491) (138.7353, -190.9294) (138.2342, -191.1898) knots 0 0 0 0 1 1 1 1
  spline S257 degree 3 poles (138.2342, -191.1898) (137.7331, -191.4502) (137.3767, -191.8867) (137.277, -192.3623) knots 0 0 0 0 1 1 1 1
  line L82 (137.277, -192.3623) -> (136.5829, -192.347)
  line L83 (136.5829, -192.347) -> (136.504, -190.9508)
  spline S258 degree 3 poles (136.504, -190.9508) (136.4991, -190.8676) (136.4905, -190.7829) (136.4504, -190.7062) knots 0 0 0 0 1 1 1 1
  spline S259 degree 3 poles (136.4504, -190.7062) (136.4103, -190.6296) (136.3402, -190.563) (136.2518, -190.5207) knots 0 0 0 0 1 1 1 1
  spline S260 degree 3 poles (136.2518, -190.5207) (136.186, -190.4891) (136.1079, -190.4718) (136.0323, -190.481) knots 0 0 0 0 1 1 1 1
  spline S261 degree 3 poles (136.0323, -190.481) (135.9945, -190.4859) (135.958, -190.4966) (135.9248, -190.5118) knots 0 0 0 0 1 1 1 1
  spline S262 degree 3 poles (135.9248, -190.5118) (135.8915, -190.5271) (135.8615, -190.5466) (135.8319, -190.5663) knots 0 0 0 0 1 1 1 1
  line L84 (135.8319, -190.5663) -> (135.2966, -190.9214)
  line L85 (135.2966, -190.9214) -> (135.2162, -192.1137)
  line L86 (135.2162, -192.1137) -> (133.7361, -192.1098)
  spline S263 degree 3 poles (133.7361, -192.1098) (133.4277, -192.1286) (133.1343, -192.2703) (132.9672, -192.4812) knots 0 0 0 0 1 1 1 1
  spline S264 degree 3 poles (132.9672, -192.4812) (132.873, -192.6001) (132.8181, -192.7384) (132.8021, -192.879) knots 0 0 0 0 1 1 1 1
  spline S265 degree 3 poles (132.8021, -192.879) (132.786, -193.0197) (132.8081, -193.1626) (132.8598, -193.2975) knots 0 0 0 0 1 1 1 1
  spline S266 degree 3 poles (132.8598, -193.2975) (132.9629, -193.5673) (133.1808, -193.801) (133.4379, -193.9917) knots 0 0 0 0 1 1 1 1
  spline S267 degree 3 poles (133.4379, -193.9917) (133.6551, -194.1528) (133.9019, -194.2867) (134.1641, -194.3951) knots 0 0 0 0 1 1 1 1
  spline S268 degree 3 poles (184.3644, -181.7042) (184.3072, -181.7021) (184.2498, -181.7032) (184.1928, -181.7073) knots 0 0 0 0 1 1 1 1
  spline S269 degree 3 poles (184.1928, -181.7073) (183.1609, -181.9463) (183.3223, -182.3642) (183.2158, -182.9775) knots 0 0 0 0 1 1 1 1
  spline S270 degree 3 poles (183.2158, -182.9775) (183.2445, -183.2215) (183.2367, -183.5508) (183.2584, -183.8669) knots 0 0 0 0 1 1 1 1
  spline S271 degree 3 poles (183.2584, -183.8669) (182.8081, -183.8947) (182.6359, -183.8492) (182.258, -183.8892) knots 0 0 0 0 1 1 1 1
  spline S272 degree 3 poles (182.258, -183.8892) (182.1006, -184.1017) (182.2375, -184.7485) (182.4445, -185.1212) knots 0 0 0 0 1 1 1 1
  spline S273 degree 3 poles (182.4445, -185.1212) (182.7792, -185.2644) (182.8517, -185.2273) (183.208, -185.2182) knots 0 0 0 0 1 1 1 1
  spline S274 degree 3 poles (183.208, -185.2182) (183.6977, -185.2488) (183.7264, -185.2388) (184.108, -185.26) knots 0 0 0 0 1 1 1 1
  spline S275 degree 3 poles (184.108, -185.26) (184.1435, -185.8767) (184.1498, -185.9165) (184.197, -186.9512) knots 0 0 0 0 1 1 1 1
  spline S276 degree 3 poles (184.197, -186.9512) (184.1919, -187.3908) (184.1986, -187.3959) (184.2304, -188.144) knots 0 0 0 0 1 1 1 1
  spline S277 degree 3 poles (184.2304, -188.144) (183.6828, -188.1911) (183.4861, -188.1839) (183.0062, -188.213) knots 0 0 0 0 1 1 1 1
  spline S278 degree 3 poles (183.0062, -188.213) (182.8873, -188.2777) (182.9813, -188.6981) (183.0158, -188.934) knots 0 0 0 0 1 1 1 1
  spline S279 degree 3 poles (183.0158, -188.934) (183.1529, -189.425) (183.1143, -189.379) (183.7285, -189.4211) knots 0 0 0 0 1 1 1 1
  line L87 (183.7285, -189.4211) -> (184.4253, -189.4019)
  spline S280 degree 3 poles (184.4253, -189.4019) (184.4431, -190.1405) (184.6181, -192.1908) (184.4671, -192.5158) knots 0 0 0 0 1 1 1 1
  spline S281 degree 3 poles (184.4671, -192.5158) (183.3716, -191.7213) (182.2011, -193.6456) (183.2991, -193.8209) knots 0 0 0 0 1 1 1 1
  spline S282 degree 3 poles (183.2991, -193.8209) (183.788, -193.8708) (184.1067, -193.8923) (184.635, -193.9853) knots 0 0 0 0 1 1 1 1
  spline S283 degree 2 poles (184.635, -193.9853) (184.6996, -194.4616) (184.7164, -194.7726) knots 0 0 0 1 1 1
  spline S284 degree 3 poles (184.7164, -194.7726) (183.8445, -195.299) (183.3568, -195.8773) (183.1814, -196.7222) knots 0 0 0 0 1 1 1 1
  spline S285 degree 3 poles (183.1814, -196.7222) (183.128, -197.543) (183.6457, -198.7232) (184.6149, -198.9876) knots 0 0 0 0 1 1 1 1
  line L88 (184.6149, -198.9876) -> (184.3632, -200.3109)
  spline S286 degree 3 poles (184.3632, -200.3109) (183.7331, -200.4934) (183.5113, -200.5128) (182.8815, -200.555) knots 0 0 0 0 1 1 1 1
  spline S287 degree 3 poles (182.8815, -200.555) (182.5615, -200.5841) (182.6889, -200.8048) (182.7564, -201.0891) knots 0 0 0 0 1 1 1 1
  spline S288 degree 3 poles (182.7564, -201.0891) (182.8568, -201.413) (182.7298, -201.5024) (183.0873, -201.6832) knots 0 0 0 0 1 1 1 1
  spline S289 degree 3 poles (183.0873, -201.6832) (183.4045, -201.7953) (183.5789, -201.8659) (183.9066, -202.058) knots 0 0 0 0 1 1 1 1
  spline S290 degree 3 poles (183.9066, -202.058) (183.9338, -202.3687) (183.9163, -202.7859) (183.9473, -203.1082) knots 0 0 0 0 1 1 1 1
  spline S291 degree 3 poles (183.9473, -203.1082) (184.1158, -203.7792) (184.5287, -203.952) (185.2606, -203.8828) knots 0 0 0 0 1 1 1 1
  spline S292 degree 3 poles (185.2606, -203.8828) (186.0534, -203.5748) (186.3323, -203.0203) (186.3836, -202.3626) knots 0 0 0 0 1 1 1 1
  spline S293 degree 2 poles (186.3836, -202.3626) (186.4825, -199.2725) (186.3742, -197.9374) knots 0 0 0 1 1 1
  line L89 (186.3742, -197.9374) -> (185.3446, -196.9253)
  line L90 (185.3446, -196.9253) -> (186.5395, -195.767)
  spline S294 degree 3 poles (186.5395, -195.767) (186.3223, -191.1919) (186.2127, -187.2566) (185.5675, -182.6824) knots 0 0 0 0 1 1 1 1
  spline S295 degree 3 poles (185.5675, -182.6824) (185.3935, -182.0988) (185.0059, -181.7976) (184.3644, -181.7042) knots 0 0 0 0 1 1 1 1
  spline S296 degree 3 poles (160.3558, -156.7499) (157.851, -157.1446) (155.5033, -158.5586) (153.908, -160.6331) knots 0 0 0 0 1 1 1 1
  spline S297 degree 3 poles (153.908, -160.6331) (152.3128, -162.7076) (151.4858, -165.4223) (151.6368, -168.0885) knots 0 0 0 0 1 1 1 1
  spline S298 degree 3 poles (151.6368, -168.0885) (151.7797, -170.6139) (152.7953, -173.0742) (154.4505, -174.9052) knots 0 0 0 0 1 1 1 1
  spline S299 degree 3 poles (154.4505, -174.9052) (156.1057, -176.7362) (158.3874, -177.9235) (160.7723, -178.1946) knots 0 0 0 0 1 1 1 1
  line L91 (160.7723, -178.1946) -> (169.7138, -178.2503)
  spline S300 degree 3 poles (169.7138, -178.2503) (173.9239, -176.4208) (178.4739, -175.4662) (183.0274, -175.4572) knots 0 0 0 0 1 1 1 1
  spline S301 degree 3 poles (183.0274, -175.4572) (188.8994, -175.4456) (194.7681, -177.0191) (199.922, -179.9867) knots 0 0 0 0 1 1 1 1
  line L92 (199.922, -179.9867) -> (207.8031, -180.4742)
  spline S302 degree 3 poles (207.8031, -180.4742) (210.4446, -180.3114) (213.0075, -179.0135) (214.7796, -176.9411) knots 0 0 0 0 1 1 1 1
  spline S303 degree 3 poles (214.7796, -176.9411) (216.5517, -174.8687) (217.512, -172.0465) (217.3936, -169.2586) knots 0 0 0 0 1 1 1 1
  spline S304 degree 3 poles (217.3936, -169.2586) (217.298, -167.0064) (216.5098, -164.7927) (215.1762, -163.0309) knots 0 0 0 0 1 1 1 1
  spline S305 degree 3 poles (215.1762, -163.0309) (213.8425, -161.269) (211.9703, -159.968) (209.9091, -159.3708) knots 0 0 0 0 1 1 1 1
  line L93 (209.9091, -159.3708) -> (201.2539, -158.7324)
  spline S306 degree 3 poles (201.2539, -158.7324) (196.2254, -161.1318) (190.6511, -162.2472) (185.1387, -161.9572) knots 0 0 0 0 1 1 1 1
  spline S307 degree 3 poles (185.1387, -161.9572) (179.7234, -161.6722) (174.3764, -160.032) (169.6609, -157.2094) knots 0 0 0 0 1 1 1 1
  line L94 (169.6609, -157.2094) -> (160.3558, -156.7499)
  spline S308 degree 3 poles (158.3161, -159.7104) (158.0653, -159.7026) (157.812, -159.8077) (157.638, -159.9984) knots 0 0 0 0 1 1 1 1
  spline S309 degree 3 poles (157.638, -159.9984) (157.464, -160.189) (157.3734, -160.4626) (157.4027, -160.7254) knots 0 0 0 0 1 1 1 1
  spline S310 degree 3 poles (157.4027, -160.7254) (157.4301, -160.9723) (157.5618, -161.2031) (157.7528, -161.3486) knots 0 0 0 0 1 1 1 1
  spline S311 degree 3 poles (157.7528, -161.3486) (157.9438, -161.4941) (158.1908, -161.5535) (158.4236, -161.5149) knots 0 0 0 0 1 1 1 1
  spline S312 degree 3 poles (158.4236, -161.5149) (158.6278, -161.4811) (158.821, -161.3728) (158.9586, -161.21) knots 0 0 0 0 1 1 1 1
  spline S313 degree 3 poles (158.9586, -161.21) (159.0962, -161.0472) (159.1765, -160.8307) (159.1758, -160.6126) knots 0 0 0 0 1 1 1 1
  spline S314 degree 3 poles (159.1758, -160.6126) (159.175, -160.3769) (159.0792, -160.1441) (158.9196, -159.979) knots 0 0 0 0 1 1 1 1
  spline S315 degree 3 poles (158.9196, -159.979) (158.7601, -159.8139) (158.5395, -159.7176) (158.3161, -159.7104) knots 0 0 0 0 1 1 1 1
  spline S316 degree 3 poles (157.7104, -173.0187) (157.4597, -173.0109) (157.2064, -173.116) (157.0323, -173.3067) knots 0 0 0 0 1 1 1 1
  spline S317 degree 3 poles (157.0323, -173.3067) (156.8583, -173.4973) (156.7678, -173.771) (156.797, -174.0338) knots 0 0 0 0 1 1 1 1
  spline S318 degree 3 poles (156.797, -174.0338) (156.8244, -174.2806) (156.9562, -174.5114) (157.1472, -174.6569) knots 0 0 0 0 1 1 1 1
  spline S319 degree 3 poles (157.1472, -174.6569) (157.3382, -174.8024) (157.5851, -174.8618) (157.8179, -174.8233) knots 0 0 0 0 1 1 1 1
  spline S320 degree 3 poles (157.8179, -174.8233) (158.0222, -174.7894) (158.2154, -174.6811) (158.353, -174.5183) knots 0 0 0 0 1 1 1 1
  spline S321 degree 3 poles (158.353, -174.5183) (158.4906, -174.3555) (158.5708, -174.139) (158.5702, -173.921) knots 0 0 0 0 1 1 1 1
  spline S322 degree 3 poles (158.5702, -173.921) (158.5694, -173.6853) (158.4735, -173.4524) (158.314, -173.2873) knots 0 0 0 0 1 1 1 1
  spline S323 degree 3 poles (158.314, -173.2873) (158.1544, -173.1222) (157.9338, -173.0259) (157.7104, -173.0187) knots 0 0 0 0 1 1 1 1